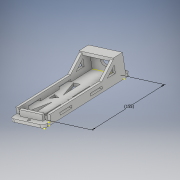
# Autodesk Inventor part: 3C_LiPoBatteryHolder
Saved by Autodesk Inventor 2018 (Build 220112000, 112)
## iProperties
Created: 2019-07-06
Part Number: 3C_LiPoBatteryHolder
Material: Generic
Document SubType Name: Modeling
Designer: Chris Taylor
Density: 1 g/cm^3
Appearance: Default
Author: Chris Taylor
Autodesk Inventor part; units mm, degrees
ref_plane "YZ Plane" through (0, 0, 0) normal (1, 0, 0) x (0, 1, 0)
ref_plane "XZ Plane" through (0, 0, 0) normal (0, 1, 0) x (-1, 0, 0)
ref_plane "XY Plane" through (0, 0, 0) normal (0, 0, 1) x (1, 0, 0)
sketch "Sketch1" plane through (0, 0, 0) normal (0, 1, 0) x (-1, 0, 0)
  line L0 (0, 0) -> (60, 0)
  line L1 (60, 0) -> (60, -170)
  line L2 (60, -170) -> (0, -170)
  line L3 (0, -170) -> (0, 0)
  dimension "d0" = 60
  dimension "d1" = 170
  constraints: 8 end point, 2 parallel, 1 horizontal, 1 perpendicular
  measures "d0" distance of L1.end L2.end
  measures "d1" distance of L0.end L1.end
extrude "Extrusion1" add sketch "Sketch1" along normal blind 5
sketch "Sketch2" plane through (0, 5, 0) normal (0, 1, 0) x (1, 0, 0)
  line L0 (-60, 0) -> (-55, 0)
  line L1 (-60, 170) -> (-60, 0) projected
  line L2 (0, 0) -> (0, 170) projected
  line L3 (-60, 170) -> (0, 170)
  line L4 (0, 170) -> (0, 162.5)
  line L5 (0, 162.5) -> (-60, 162.5)
  line L6 (-60, 162.5) -> (-60, 170)
  line L7 (-60, 0) -> (0, 0) projected
  line L8 (-60, 0) -> (0, 0)
  line L9 (0, 0) -> (0, 7.5)
  line L10 (0, 7.5) -> (-60, 7.5)
  line L11 (-60, 7.5) -> (-60, 0)
  line L12 (0, 170) -> (-60, 170) projected
  line L13 (-60, 0) -> (-55, 0)
  line L14 (-55, 0) -> (-55, 170)
  line L15 (-55, 170) -> (-60, 170)
  line L16 (-60, 170) -> (-60, 0)
  line L17 (0, 0) -> (-5, 0)
  line L18 (-5, 0) -> (-5, 170)
  line L19 (-5, 170) -> (0, 170)
  line L20 (0, 170) -> (0, 0)
  line L21 (-60, 0) -> (0, 0)
  line L22 (0, 0) -> (0, -5)
  line L23 (0, -5) -> (-60, -5)
  line L24 (-60, -5) -> (-60, 0)
  line L25 (-60, 170) -> (0, 170)
  line L26 (0, 170) -> (0, 175)
  line L27 (0, 175) -> (-60, 175)
  line L28 (-60, 175) -> (-60, 170)
  dimension "d5" = 7.5
  dimension "d6" = 7.5
  dimension "d7" = 5
  dimension "d8" = 5
  dimension "d10" = 5
  dimension "d11" = 5
  constraints: 50 end point, 12 parallel, 7 horizontal, 6 perpendicular, 4 point on line
  measures "d5" distance of L3.end L4.end
  measures "d6" distance of L9.end L8.end
  measures "d7" distance of L15.end L14.end
  measures "d8" distance of L18.end L19.end
  measures "d10" distance of L21.end L22.end
  measures "d11" distance of L26.end L25.end
extrude "Extrusion2" add sketch "Sketch2" against normal blind 5 contours L0 L7 L22 L23 L24 | L28 L27 L26 L3
sketch "Sketch3" plane through (0, 5, 0) normal (0, 1, 0) x (1, 0, 0)
  line L0 (0, -5) -> (-60, -5) projected
  line L1 (0, -5) -> (0, 175) projected
  line L2 (-60, -10) -> (0, -10)
  line L3 (0, -5) -> (0, 5)
  line L4 (-60, 5) -> (-60, -5)
  line L5 (-55, 175) -> (-60, 175)
  line L6 (-60, 175) -> (-60, 5)
  line L7 (-5, 175) -> (0, 175)
  line L8 (-60, 175) -> (-60, -5) projected
  line L9 (-60, 175) -> (-1, 175)
  line L10 (-1, 165) -> (-60, 165)
  line L11 (-60, 165) -> (-60, 175)
  line L12 (-55, 165) -> (-5, 165)
  line L13 (-5, 160) -> (-55, 160)
  line L14 (-55, 5) -> (-55, 160)
  line L15 (-5, 5) -> (-5, 160)
  line L16 (-50, 5) -> (-10, 5)
  line L17 (-10, 5) -> (-10, 5)
  line L18 (-10, 5) -> (-50, 5)
  line L19 (-50, 5) -> (-50, 5)
  line L20 (-60, 5) -> (-55, 5)
  line L21 (-5, 5) -> (0, 5)
  line L22 (0, 5) -> (0, 165)
  line L23 (-60, -5) -> (-60, -10)
  line L24 (0, -5) -> (0, -10)
  line L25 (-50, 5) -> (-50, 0)
  line L26 (-50, 0) -> (-10, 0)
  line L27 (-10, 0) -> (-10, 5)
  point P0 (0, 0)
  dimension "d15" = 5
  dimension "d16" = 5
  dimension "d17" = 10
  dimension "d18" = 5
  dimension "d19" = 40
  dimension "d89" = 155
  dimension "d90" = 5
  dimension "d91" = 10
  constraints: 50 end point, 7 parallel, 5 horizontal, 4 perpendicular, 4 point on line, 2 collinear
  measures "d15" distance of L5.end L5.start
  measures "d16" distance of L7.start L7.end
  measures "d17" distance of L9.end L10.start
  measures "d18" distance of L12.end L13.start
  measures "d19" distance of L18.end L17.end
  measures "d89" distance between parallel lines of L18 L13
  measures "d90" distance of L18.end L25.end
  measures "d91" distance from line of L2 point (0, 0)
sketch "Sketch4" plane through (0, 5, 0) normal (0, 1, 0) x (1, 0, 0)
  line L0 (-60, 175) -> (-60, -5) projected
  line L1 (-60, 5) -> (-55, 5)
  line L2 (-55, 5) -> (-55, 160)
  line L3 (-55, 160) -> (-5, 160)
  line L4 (-5, 160) -> (-5, 5)
  line L5 (-5, 5) -> (0, 5)
  line L6 (0, -5) -> (0, 175) projected
  line L7 (0, 165) -> (-60, 165)
  line L8 (-60, 165) -> (-60, 5)
  point P0 (0, 0)
  constraints: 14 end point, 5 point on line, 3 perpendicular, 1 horizontal, 1 parallel
extrude "Extrusion3" add sketch "Sketch3" along normal blind 10 contours L16 L27 L26 L25
extrude "Extrusion4" add sketch "Sketch4" along normal blind 10
sketch "Sketch5" plane through (0, 0, 5) normal (1, 0, 0) x (0, 0, -1)
  line L0 (180, 5) -> (170, 5) projected
  line L1 (170, 5) -> (165, 5)
  line L2 (165, 5) -> (165, 32)
  line L3 (165, 32) -> (170, 32)
  line L4 (170, 32) -> (170, 5)
  point P0 (5, 0)
  dimension "d25" = 5
  dimension "d26" = 27
  constraints: 8 end point, 2 parallel, 1 horizontal, 1 perpendicular
  measures "d25" distance of L2.end L3.end
  measures "d26" distance of L1.end L2.end
sketch "Sketch6" plane through (0, 5, 0) normal (0, 1, 0) x (1, 0, 0)
  point P0 (0, 0)
extrude "Extrusion5" add sketch "Sketch5" against normal blind 60
sketch "Sketch7" plane through (0, 0, 5) normal (1, 0, 0) x (0, 0, -1)
  line L0 (165, 32) -> (170, 32) projected
  line L1 (170, 32) -> (150, 32)
  line L2 (150, 32) -> (150, 35.5)
  line L3 (150, 35.5) -> (170, 35.5)
  line L4 (170, 35.5) -> (170, 32)
  point P0 (5, 0)
  dimension "d29" = 20
  dimension "d30" = 3.5
  constraints: 8 end point, 2 parallel, 1 horizontal, 1 perpendicular
  measures "d29" distance of L2.end L3.end
  measures "d30" distance of L1.end L2.end
extrude "Extrusion6" add sketch "Sketch7" against normal blind 60
sketch "Sketch8" plane through (-55, 5, -160) normal (0, 0, 1) x (1, 0, 0)
  point P0 (55, -5)
sketch "Sketch9" plane through (0, 0, 5) normal (1, 0, 0) x (0, 0, -1)
  line L0 (150, 35.5) -> (170, 35.5) projected
  line L1 (170, 35.5) -> (170, 5) projected
  line L2 (150, 35.5) -> (170, 35.5)
  line L3 (170, 35.5) -> (170, 27)
  line L4 (170, 27) -> (150, 27)
  line L5 (150, 27) -> (150, 35.5)
  point P0 (5, 0)
  constraints: 8 end point, 2 parallel, 1 horizontal, 1 perpendicular, 1 point on line
extrude "Extrusion7" add sketch "Sketch9" against normal blind 5
sketch "Sketch10" plane through (0, 0, 5) normal (1, 0, 0) x (0, 0, -1)
  line L0 (150, 35.5) -> (150, 27) projected
  line L1 (150, 27) -> (132.8622, 15)
  line L2 (10, 15) -> (165, 15) projected
  line L3 (150, 27) -> (170.9214, 27) construction
  line L4 (150, 35.5) -> (170, 35.5) projected
  line L5 (150, 35.5) -> (120.723, 15)
  line L6 (150, 35.5) -> (185.7407, 35.5) construction
  line L7 (132.8622, 15) -> (120.723, 15)
  line L8 (150, 35.5) -> (150, 27)
  point P0 (5, 0)
  dimension "d35" = 145
  dimension "d36" = 145
  constraints: 12 end point, 2 collinear, 2 equal length, 2 horizontal, 2 point on line
  measures "d35" angle of L1 L3
  measures "d36" angle of L5 L6
extrude "Extrusion8" add sketch "Sketch10" against normal blind 5
sketch "Sketch11" plane through (0, 0, 5) normal (1, 0, 0) x (0, 0, -1)
  point P0 (5, 0)
sketch "Sketch12" plane through (-60, 0, -175) normal (-1, 0, 0) x (0, 0, 1)
  line L0 (10, 35.5) -> (10, 5) projected
  line L1 (15, 27) -> (30, 27) projected
  line L2 (10, 35.5) -> (30, 35.5)
  line L3 (30, 35.5) -> (30, 27)
  line L4 (30, 27) -> (10, 27)
  line L5 (10, 27) -> (10, 35.5)
  point P0 (175, 0)
  constraints: 8 end point, 2 parallel, 1 horizontal, 1 perpendicular
extrude "Extrusion9" add sketch "Sketch12" against normal blind 5
sketch "Sketch13" plane through (-60, 0, -175) normal (-1, 0, 0) x (0, 0, 1)
  line L0 (30, 27) -> (47.1378, 15)
  line L1 (15, 15) -> (170, 15) projected
  line L2 (30, 27) -> (50.9214, 27) construction
  line L3 (30, 32) -> (30, 35.5) projected
  line L4 (30, 35.5) -> (59.277, 15)
  line L5 (30, 35.5) -> (65.7407, 35.5) construction
  line L6 (59.277, 15) -> (47.1378, 15)
  line L7 (30, 27) -> (15, 27) projected
  line L8 (30, 35.5) -> (30, 27) projected
  line L9 (30, 27) -> (30, 35.5)
  point P0 (175, 0)
  dimension "d41" = 35
  dimension "d42" = 35
  constraints: 12 end point, 2 collinear, 2 equal length, 2 horizontal, 2 point on line
  measures "d41" angle of L0 L2
  measures "d42" angle of L4 L5
extrude "Extrusion10" add sketch "Sketch13" against normal blind 5
sketch "Sketch14" plane through (0, 0, 5) normal (1, 0, 0) x (0, 0, -1)
  line L0 (107.1526, 5) -> (92.1526, 5)
  line L1 (92.1526, 5) -> (92.1526, 7)
  line L2 (92.1526, 7) -> (107.1526, 7)
  line L3 (107.1526, 7) -> (107.1526, 5)
  line L4 (20, 5) -> (35, 5)
  line L5 (35, 5) -> (35, 7)
  line L6 (35, 7) -> (20, 7)
  line L7 (20, 7) -> (20, 5)
  point P0 (5, 0)
  point P1 (10, 5)
  point P2 (120.723, 15)
  dimension "d45" = 10
  dimension "d47" = 15
  dimension "d48" = 15
  constraints: 16 end point, 4 parallel, 2 horizontal, 2 perpendicular, 1 point on line
  measures "d45" distance of point (10, 5) L4.start
  measures "d47" distance of L1.end L2.end
  measures "d48" distance of L6.end L5.end
extrude "Extrusion11" cut sketch "Sketch14" against normal through all
sketch "Sketch15" plane through (0, 5, -165) normal (0, 0, -1) x (-1, 0, 0)
  circle A0 centre (30, 16) radius 7.5
  point P0 (0, -5)
  point P1 (0, 30.5)
  dimension "d53" = 15
  constraints: 1 centre point
  measures "d53" diameter of A0
extrude "Extrusion12" cut sketch "Sketch15" against normal blind 5
sketch "Sketch16" plane through (0, 0, 5) normal (1, 0, 0) x (0, 0, -1)
  line L0 (165, 27) -> (150, 27) projected
  line L1 (165, 15) -> (165, 27) projected
  line L2 (150, 27) -> (165, 27)
  line L3 (165, 27) -> (165, 15)
  line L4 (165, 15) -> (150, 15)
  line L5 (150, 15) -> (150, 27)
  point P0 (5, 0)
  constraints: 8 end point, 2 parallel, 1 horizontal, 1 perpendicular
extrude "Extrusion13" add sketch "Sketch16" against normal blind 5
sketch "Sketch17" plane through (-60, 0, -175) normal (-1, 0, 0) x (0, 0, 1)
  line L0 (30, 27) -> (15, 27) projected
  line L1 (47.1378, 15) -> (30, 15) projected
  line L2 (15, 27) -> (30, 27)
  line L3 (30, 27) -> (30, 15)
  line L4 (30, 15) -> (15, 15)
  line L5 (15, 15) -> (15, 27)
  point P0 (175, 0)
  constraints: 8 end point, 2 parallel, 1 horizontal, 1 perpendicular
extrude "Extrusion14" add sketch "Sketch17" against normal blind 5
fillet "Fillet1" radius 7 4 edges at (0, 2.5, -175) (-60, 2.5, -175) (0, 2.5, 5) (-60, 2.5, 5)
sketch "Sketch19" plane through (0, 5, 0) normal (0, 1, 0) x (1, 0, 0)
  line L0 (-50, 5) -> (-50, 5) projected
  line L1 (-50, 17) -> (-38, 17)
  line L2 (-38, 17) -> (-38, 53)
  line L3 (-38, 53) -> (-50, 17)
  line L4 (-10, 22) -> (-22, 22)
  line L5 (-22, 22) -> (-22, 58)
  line L6 (-22, 58) -> (-10, 22)
  line L7 (-38, 78) -> (-38, 114)
  line L8 (-38, 114) -> (-50, 114)
  line L9 (-50, 114) -> (-38, 78)
  line L10 (-22, 78) -> (-22, 114)
  line L11 (-22, 114) -> (-10, 114)
  line L12 (-10, 114) -> (-22, 78)
  point P0 (0, 0)
  dimension "d67" = 12
  dimension "d68" = 12
  dimension "d69" = 36
  dimension "d71" = 12
  dimension "d72" = 36
  dimension "d73" = 12
  dimension "d74" = 20
  dimension "d75" = 36
  dimension "d76" = 12
  constraints: 24 end point, 4 perpendicular, 1 horizontal, 1 point on line, 1 vertical
  measures "d67" distance of L0.start L1.start
  measures "d68" distance of L1.start L1.end
  measures "d69" distance of L1.end L2.end
  measures "d71" distance of L4.start L4.end
  measures "d72" distance of L7.start L7.end
  measures "d73" distance of L7.end L8.end
  measures "d74" distance of L5.end L10.start
  measures "d75" distance of L10.start L10.end
  measures "d76" distance of L10.end L11.end
extrude "Extrusion16" cut sketch "Sketch19" against normal blind 5
sketch "Sketch20" plane through (0, 5, 0) normal (0, 1, 0) x (1, 0, 0)
  line L0 (-38, 17) -> (-50, 17) projected
  line L1 (-50, 114) -> (-38, 78) projected
  line L2 (-38, 78) -> (-38, 114) projected
  line L3 (-38, 68) -> (-50, 74)
  line L4 (-50, 62) -> (-38, 68)
  line L5 (-50, 74) -> (-50, 62)
  line L6 (-22, 68) -> (-10, 62)
  line L7 (-10, 74) -> (-22, 68)
  line L8 (-10, 62) -> (-10, 74)
  point P0 (0, 0)
  constraints: 12 end point, 1 vertical
extrude "Extrusion17" cut sketch "Sketch20" against normal blind 5
sketch "Sketch21" plane through (-60, 5, -5) normal (-1, 0, 0) x (0, 0, 1)
  line L0 (-17, 0) -> (-53, 0) projected
  line L1 (-7, 2) -> (-31, 2)
  line L2 (-31, 2) -> (-31, 0)
  line L3 (-31, 0) -> (-7, 0)
  line L4 (-7, 0) -> (-7, 2)
  line L5 (-79, 2) -> (-103, 2)
  line L6 (-103, 2) -> (-103, 0)
  line L7 (-103, 0) -> (-79, 0)
  line L8 (-79, 0) -> (-79, 2)
  point P0 (5, -5)
  dimension "d84" = 24
  dimension "d85" = 24
  constraints: 16 end point, 4 parallel, 3 point on line, 2 horizontal, 2 perpendicular
  measures "d84" distance of L3.end L2.end
  measures "d85" distance of L7.end L6.end
extrude "Extrusion18" cut sketch "Sketch21" against normal through all
sketch "Sketch22" plane through (0, 5, 0) normal (0, 1, 0) x (1, 0, 0)
  point P0 (0, 0)
sketch "Sketch24" plane through (0, 5, 0) normal (0, 1, 0) x (1, 0, 0)
  point P0 (0, 0)
sketch "Sketch25" plane through (0, 5, 0) normal (0, 1, 0) x (1, 0, 0)
  point P0 (0, 0)
sketch "Sketch26" plane through (0, 5, 0) normal (0, 1, 0) x (1, 0, 0)
  arc A0 (-60, 2) -> (-53, -5) centre (-53, 2) ccw projected
  line L0 (-60, 2) -> (0, 2)
  line L1 (0, 2) -> (0, -10)
  line L2 (0, -10) -> (-60, -10)
  line L3 (-60, -10) -> (-60, 2)
  point P0 (0, 0)
  dimension "d93" = 12
  constraints: 8 end point, 3 perpendicular, 1 horizontal, 1 tangent
  measures "d93" distance of L0.end L1.end
extrude "Extrusion19" add sketch "Sketch26" against normal blind 5
sketch "Sketch27" plane through (0, 5, 0) normal (0, 1, 0) x (1, 0, 0)
  point P0 (0, 0)
sketch "Sketch28" plane through (-60, 5, 10) normal (0, 0, 1) x (1, 0, 0)
  point P0 (60, -5)
sketch "Sketch29" plane through (0, 5, 0) normal (0, 1, 0) x (1, 0, 0)
  line L0 (-30, -10) -> (-30, -5)
  circle A0 centre (-30, -5) radius 2.5
  arc A1 (-53, 175) -> (-60, 168) centre (-53, 168) ccw projected
  line L1 (-7, 175) -> (-53, 175) projected
  line L2 (-30, 175) -> (-30, 170)
  circle A2 centre (-30, 170) radius 2.5
  point P0 (0, 0)
  point P1 (-60, -10)
  dimension "d96" = 30
  dimension "d97" = 5
  dimension "d98" = 5
  dimension "d102" = 5
  constraints: 4 end point, 2 centre point, 2 coincident, 1 midpoint
  measures "d96" distance of point (-60, -10) L0.start
  measures "d97" distance of L0.start L0.end
  measures "d98" diameter of A0
  measures "d102" distance of L2.start L2.end
extrude "Extrusion20" cut sketch "Sketch29" along normal mid plane 10
fillet "Fillet2" radius 7 2 edges at (-60, 2.5, 10) (0, 2.5, 10)
sketch "Sketch30" plane through (0, 5, 0) normal (0, 1, 0) x (1, 0, 0)
  line L0 (-22, 22) -> (-10, 22) projected
  line L1 (-24, 58) -> (-10, 58)
  line L2 (-10, 58) -> (-10, 22)
  line L3 (-10, 22) -> (-24, 22)
  line L4 (-24, 22) -> (-24, 58)
  point P0 (0, 0)
  constraints: 8 end point, 2 parallel, 1 horizontal, 1 perpendicular
extrude "Extrusion21" add sketch "Sketch30" against normal blind 5
sketch "Sketch31" plane through (0, 5, 0) normal (0, 1, 0) x (1, 0, 0)
  point P0 (0, 0)
sketch "Sketch32" plane through (0, 5, 0) normal (0, 1, 0) x (1, 0, 0)
  line L0 (-38, 53) -> (-50, 17) projected
  line L1 (-50, 17) -> (-38, 17) projected
  line L2 (-22, 53) -> (-22, 17)
  line L3 (-22, 53) -> (-10, 17)
  line L4 (-22, 17) -> (-10, 17)
  point P0 (0, 0)
  constraints: 6 end point
extrude "Extrusion22" add sketch "Sketch32" against normal blind 2
sketch "Sketch33" plane through (0, 5, 0) normal (0, 1, 0) x (1, 0, 0)
  point P0 (0, 0)
sketch "Sketch34" plane through (0, 5, 0) normal (0, 1, 0) x (1, 0, 0)
  line L0 (-5, 160) -> (-55, 160) projected
  line L1 (-50, 5) -> (-10, 5) projected
  point P0 (0, 0)
  dimension "d111" = 155
  measures "d111" distance between parallel lines of L0 L1
sketch "Sketch35" plane through (-55, 5, -160) normal (0, 0, 1) x (1, 0, 0)
  point P0 (55, -5)
sketch "Sketch37" plane through (0, 5, 0) normal (0, 1, 0) x (1, 0, 0)
  line L0 (-22, 68) -> (-10, 62) projected
  line L1 (-38, 17) -> (-50, 17) projected
  line L2 (-10, 74) -> (-10, 62) projected
  line L3 (-38, 53) -> (-38, 17) projected
  line L4 (-22, 53) -> (-22, 17)
  line L5 (-10, 17) -> (-22, 53)
  line L6 (-22, 17) -> (-10, 17)
  point P0 (0, 0)
  constraints: 6 end point, 1 horizontal
extrude "Extrusion23" cut sketch "Sketch37" against normal blind 10
sketch "Sketch38" plane through (0, 5, -5) normal (1, 0, 0) x (0, 0, -1)
  line L0 (31, 2) -> (7, 2) projected
  line L1 (31, 0) -> (31, 2) projected
  line L2 (7, 2) -> (31, 2)
  line L3 (31, 2) -> (31, 0)
  line L4 (31, 0) -> (7, 0)
  line L5 (7, 0) -> (7, 2)
  line L6 (103, 0) -> (79, 0) projected
  line L7 (79, 2) -> (103, 2)
  line L8 (103, 2) -> (103, 0)
  line L9 (103, 0) -> (79, 0)
  line L10 (79, 0) -> (79, 2)
  point P0 (-5, -5)
  constraints: 16 end point, 4 parallel, 2 horizontal, 2 perpendicular
extrude "Extrusion24" add sketch "Sketch38" against normal blind 5
sketch "Sketch39" plane through (-60, 5, -5) normal (-1, 0, 0) x (0, 0, 1)
  line L0 (-103, 2) -> (-103, 0) projected
  line L1 (-79, 0) -> (-79, 2) projected
  line L2 (-103, 2) -> (-79, 2)
  line L3 (-79, 2) -> (-79, 0)
  line L4 (-79, 0) -> (-103, 0)
  line L5 (-103, 0) -> (-103, 2)
  line L6 (-31, 2) -> (-7, 2) projected
  line L7 (-7, 0) -> (-31, 0) projected
  line L8 (-31, 2) -> (-7, 2)
  line L9 (-7, 2) -> (-7, 0)
  line L10 (-7, 0) -> (-31, 0)
  line L11 (-31, 0) -> (-31, 2)
  point P0 (5, -5)
  constraints: 16 end point, 4 parallel, 2 horizontal, 2 perpendicular
extrude "Extrusion25" add sketch "Sketch39" against normal blind 5
sketch "Sketch40" plane through (0, 5, -5) normal (1, 0, 0) x (0, 0, -1)
  line L0 (0, 0) -> (0, 10) projected
  line L1 (0, 0) -> (20, 0)
  line L2 (0, 0) -> (155, 0) projected
  line L3 (20, 0) -> (70, 0)
  line L4 (70, 0) -> (85, 0)
  line L5 (20, 0) -> (45, 0)
  line L6 (45, 0) -> (45, 4)
  line L7 (45, 4) -> (20, 4)
  line L8 (20, 4) -> (20, 0)
  line L9 (85, 0) -> (110, 0)
  line L10 (110, 0) -> (110, 4)
  line L11 (110, 4) -> (85, 4)
  line L12 (85, 4) -> (85, 0)
  point P0 (-5, -5)
  dimension "d118" = 20
  dimension "d119" = 50
  dimension "d120" = 15
  dimension "d121" = 25
  dimension "d122" = 4
  dimension "d123" = 25
  dimension "d124" = 4
  constraints: 22 end point, 4 parallel, 3 point on line, 2 horizontal, 2 perpendicular
  measures "d118" distance of L0.start L1.end
  measures "d119" distance of L1.end L3.end
  measures "d120" distance of L3.end L4.end
  measures "d121" distance of L7.end L6.end
  measures "d122" distance of L6.end L5.end
  measures "d123" distance of L11.end L10.end
  measures "d124" distance of L10.end L9.end
extrude "Extrusion26" cut sketch "Sketch40" against normal through all
sketch "Sketch41" plane through (-55, 5, -160) normal (0, 0, 1) x (1, 0, 0)
  point P0 (55, -5)
sketch "Sketch42" plane through (-60, 35.5, -165) normal (0, 1, 0) x (1, 0, 0)
  line L0 (0, 0) -> (60, 0)
  line L1 (60, 0) -> (60, -20)
  line L2 (60, -20) -> (0, -20)
  line L3 (0, -20) -> (0, 0)
  point P0 (60, -165)
  constraints: 8 end point, 2 parallel, 1 horizontal, 1 perpendicular
extrude "Extrusion27" add sketch "Sketch42" along normal blind 2
sketch "Sketch43" plane through (0, 5, -5) normal (1, 0, 0) x (0, 0, -1)
  point P0 (-5, -5)
sketch "Sketch44" plane through (0, 5, 0) normal (0, 1, 0) x (1, 0, 0)
  point P0 (0, 0)
body "Solid1"
